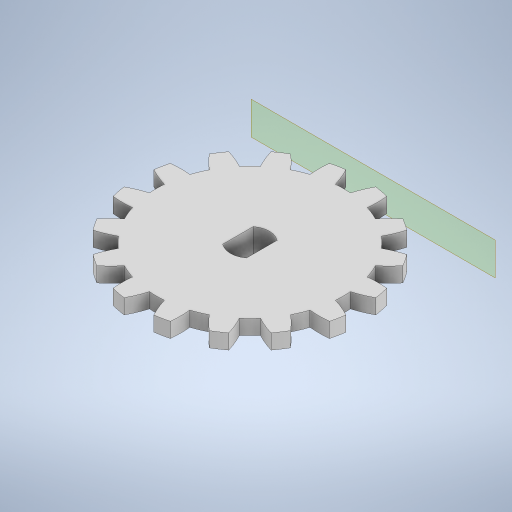
# Autodesk Inventor part: Adapter Stepper
Saved by Autodesk Inventor 2024 (Build 280153000, 153)
## iProperties
Created: 2024-01-09
Part Number: Adapter Stepper
Material: Generisch
Document SubType Name: Modeling
Designer: mariu
Density: 1 g/cm^3
Appearance: Vorgabe
Author: mariu
Autodesk Inventor part; units mm, degrees
ref_plane "YZ Plane" through (0, 0, 0) normal (1, 0, 0) x (0, 1, 0)
ref_plane "XY Plane" through (0, 0, 0) normal (0, 0, 1) x (1, 0, 0)
sketch "Skizze1" plane through (0, 0, 0) normal (0, 0, 1) x (1, 0, 0)
  circle A0 centre (0, 0) radius 2.6
  circle A1 centre (0, 0) radius 15
  line L0 (-1.6, 2.0494) -> (-1.6, -2.0494)
  line L1 (1.6, -2.0494) -> (1.6, 2.0494)
  dimension "d0" = 5.2
  dimension "d1" = 30
  dimension "d2" = 3.2
  constraints: 4 end point, 4 point on circle, 2 centre point, 2 coincident, 1 horizontal alignment, 1 parallel, 1 vertical
  measures "d0" diameter of A0
  measures "d1" diameter of A1
  measures "d2" distance between parallel lines of L1 L0
extrude "Extrusion1" add sketch "Skizze1" along normal blind 4 contours A0 L1 | L0 A0 | A1
sketch "Skizze3" plane through (0, 0, 0) normal (0, 0, -1) x (-1, 0, 0)
  circle A0 centre (0, 0) radius 5
  circle A1 centre (0, 0) radius 15
  dimension "d8" = 10
  dimension "d9" = 30
  constraints: 2 centre point, 2 coincident
  measures "d8" diameter of A0
  measures "d9" diameter of A1
extrude "Extrusion3" cut sketch "Skizze3" against normal blind 2
sketch "Skizze4" plane through (0, 0, 2) normal (0, 0, -1) x (-1, 0, 0)
  circle A0 centre (0, 0) radius 12.5 construction
  circle A1 centre (0, 0) radius 15 projected
  line L0 (-15, 0) -> (-12.5, 0)
  arc A2 (-12.4599, -1) -> (-14.8661, -2) centre (-8.8919, -12.9799) ccw
  arc A3 (-14.8661, 2) -> (-12.4599, 1) centre (-8.8919, 12.9799) ccw
  arc A4 (-14.8661, 2) -> (-14.8661, -2) centre (0, 0) ccw
  arc A5 (-12.4599, 1) -> (-12.4599, -1) centre (0, 0) ccw
  circle A6 centre (0, 0) radius 15 projected
  point P0 (-13.75, 0)
  dimension "d12" = 25
  dimension "d13" = 12.5
  dimension "d14" = 4
  dimension "d15" = 2
  constraints: 14 point on circle, 5 centre point, 2 concentric, 2 end point, 1 coincident, 1 horizontal, 1 horizontal alignment, 1 midpoint, 1 other
  measures "d12" diameter of A0
  measures "d13" radius of A2
  measures "d14" distance of A3.start A1.end
  measures "d15" distance of A3.end A0.end
extrude "Extrusion4" cut sketch "Skizze4" against normal blind 2 contours A3 A5 L0 A1 | A1 L0 A5 A2
pattern_circular "Runde Anordnung1" count 16 over 360 about axis through (0, 0, 0) along (0, 0, 1) of "Extrusion4"
ref_plane "Arbeitsebene1" through (0, 16.5, 0) normal (0, 1, 0) x (-1, 0, 0)
